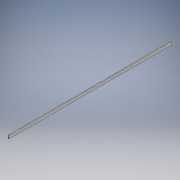
# Autodesk Inventor part: Boden_airline_eckig
Saved by Autodesk Inventor 2018 (Build 220112000, 112)
## iProperties
Created: 2020-03-29
Part Number: Boden_airline_eckig
Material: Generisch
Document SubType Name: Blech
Designer: wepet
Density: 1 g/cm^3
Sheet Metal Rule: Standard_mm
Appearance: Vorgabe
Author: wepet
Autodesk Inventor part; units mm, degrees
ref_plane "YZ Plane" through (0, 0, 0) normal (1, 0, 0) x (0, 1, 0)
ref_plane "XZ Plane" through (0, 0, 0) normal (0, 1, 0) x (-1, 0, 0)
ref_plane "XY Plane" through (0, 0, 0) normal (0, 0, 1) x (1, 0, 0)
sketch "Skizze2" plane through (0, 0, 0) normal (0, 1, 0) x (-1, 0, 0)
  line L0 (0, 0) -> (1, 0) construction
  line L1 (1, 0) -> (1, -3.4) construction
  line L2 (1, -3.4) -> (0, -3.4) construction
  line L3 (0, -3.4) -> (0, 0) construction
  line L4 (0.7, -3.1) -> (0.7, -0.3) construction
  line L5 (0.7, -0.3) -> (0.3, -0.3) construction
  line L6 (0.3, -0.3) -> (0.3, -3.1) construction
  line L7 (0.3, -3.1) -> (0.7, -3.1) construction
  line L8 (1, -1.7) -> (0, -1.7) construction
  line L9 (1, -1.2) -> (0.7, -1.2)
  line L10 (1, -2.2) -> (0.7, -2.2)
  line L11 (1, -1.2) -> (1, 0)
  line L12 (0, 0) -> (0, -3.4)
  line L13 (1, -3.4) -> (1, -2.2)
  line L14 (0.7, -2.2) -> (0.7, -3.1)
  line L15 (0.3, -3.1) -> (0.3, -0.3)
  line L16 (0.7, -0.3) -> (0.7, -1.2)
  line L17 (0.7, -0.3) -> (0.3, -0.3)
  line L18 (1, 0) -> (0, 0)
  line L19 (0.3, -3.1) -> (0.7, -3.1)
  line L20 (1, -3.4) -> (0, -3.4)
  dimension "d0" = 1
  dimension "d1" = 3.4
  dimension "d2" = 0.3
  dimension "d3" = 0.5
  dimension "d4" = 0.5
  constraints: 42 end point, 8 collinear, 5 parallel, 4 perpendicular, 4 point on line, 2 midpoint, 1 horizontal, 3 other
  measures "d0" distance of L1.end L2.end
  measures "d1" distance of L0.end L1.end
  measures "d2" distance between parallel lines of L1 L4
  measures "d3" distance between parallel lines of L10 L8
  measures "d4" distance between parallel lines of L8 L9
extrude "Extrusion1" add sketch "Skizze2" along normal blind 197.5
equation "\"Biegeradius\" = Stärke"
equation "\"BreiteBiegungsfreistellung\" = Stärke"
equation "\"TiefeBiegungsfreistellung\" = 0.5 * Stärke"
equation "\"GrößeEckenfreistellung\" = 4 * Stärke"
equation "\"MinimalRest\" = 2 * Stärke"
equation "\"Übergangsradius\" = Biegeradius"
equation "\"JacobiRadiusGröße\" = Biegeradius"
equation "\"Abstandsgröße\" = Stärke"
equation "\"Stärke\" = 0.5"
